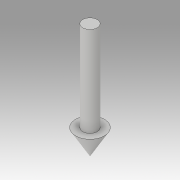
# Autodesk Inventor part: Arrow
Saved by Autodesk Inventor 2019.4 (Build 234330000, 330)
## iProperties
Created: 2021-05-25
Part Number: Arrow
Material: Generic
Document SubType Name: Modeling
Designer: D. HA
Density: 1 g/cm^3
Appearance: Default
Author: D. HA
Autodesk Inventor part; units mm, degrees
ref_plane "YZ Plane" through (0, 0, 0) normal (1, 0, 0) x (0, 1, 0)
ref_plane "XZ Plane" through (0, 0, 0) normal (0, 1, 0) x (-1, 0, 0)
ref_plane "XY Plane" through (0, 0, 0) normal (0, 0, 1) x (1, 0, 0)
sketch "Sketch1" plane through (0, 0, 0) normal (0, 0, 1) x (1, 0, 0)
  line L0 (0, 0) -> (8, 0)
  line L1 (8, 0) -> (8, -100)
  line L2 (8, -100) -> (16, -100)
  line L3 (16, -100) -> (0, -127.7128)
  line L4 (0, -127.7128) -> (0, 0)
  dimension "d0" = 8
  dimension "d1" = 100
  dimension "d3" = 16
  dimension "d4" = 30
  constraints: 10 end point, 2 perpendicular, 1 horizontal, 1 parallel
  measures "d0" distance of L0.start L0.end
  measures "d1" distance of L0.end L1.end
  measures "d3" horizontal distance of L0.start L2.end
  measures "d4" angle of L4 L3
revolve "Revolution1" add sketch "Sketch1" angle 360 about axis through (0, -127.7128, 0) along (0, 1, 0)
body "Solid1"
